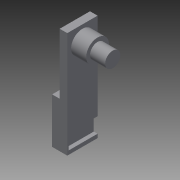
# Autodesk Inventor part: rotator_Base
Saved by Autodesk Inventor 2015 (Build 190159000, 159)
## iProperties
Created: 2015-04-10
Part Number: rotator_Base
Material: Generic
Document SubType Name: Modeling
Designer: WASHHSST
Density: 1 g/cm^3
Appearance: Default
Author: WASHHSST
Autodesk Inventor part; units mm, degrees
ref_plane "YZ Plane" through (0, 0, 0) normal (1, 0, 0) x (0, 1, 0)
ref_plane "XZ Plane" through (0, 0, 0) normal (0, 1, 0) x (-1, 0, 0)
ref_plane "XY Plane" through (0, 0, 0) normal (0, 0, 1) x (1, 0, 0)
sketch "Sketch1" plane through (0, 0, 0) normal (0, 1, 0) x (-1, 0, 0)
  line L0 (0, 0) -> (25.4, 0)
  line L1 (25.4, 0) -> (25.4, -50.8)
  line L2 (25.4, -50.8) -> (0, -50.8)
  line L3 (0, -50.8) -> (0, 0)
  dimension "d0" = 25.4
  dimension "d1" = 50.8
  constraints: 8 end point, 2 parallel, 1 horizontal, 1 perpendicular
  measures "d0" distance of L1.end L2.end
  measures "d1" distance of L0.end L1.end
extrude "Extrusion1" add sketch "Sketch1" along normal blind 25.4
sketch "Sketch2" plane through (0, 25.4, 0) normal (0, 1, 0) x (1, 0, 0)
  line L0 (-25.4, 0) -> (0, 0) projected
  line L1 (-12.7, 0) -> (-12.7, 50.8)
  line L2 (0, 50.8) -> (-25.4, 50.8) projected
  line L3 (0, 0) -> (0, 50.8) projected
  dimension "d4" = 12.7
  constraints: 2 end point, 2 midpoint, 1 vertical
  measures "d4" distance between parallel lines of L3 L1
extrude "Extrusion2" add sketch "Sketch2" along normal blind 101.6
sketch "Sketch3" plane through (0, 0, 0) normal (1, 0, 0) x (0, 0, -1)
  circle A0 centre (25.4, 101.6) radius 12.7
  line L0 (0, 0) -> (0, 127) projected
  line L1 (0, 127) -> (50.8, 127) projected
  dimension "d7" = 25.4
  dimension "d8" = 25.4
  dimension "d9" = 25.4
  constraints: 1 centre point
  measures "d7" diameter of A0
  measures "d8" distance from line of L0 A0.centre
  measures "d9" distance from line of L1 A0.centre
extrude "Extrusion3" add sketch "Sketch3" along normal blind 50.8
sketch "Sketch4" plane through (0, 0, 0) normal (0, -1, 0) x (1, 0, 0)
  line L0 (0, 0) -> (-25.4, 0)
  line L1 (-25.4, 0) -> (-25.4, -50.8)
  line L2 (-25.4, -50.8) -> (0, -50.8)
  line L3 (0, -50.8) -> (0, 0)
  constraints: 8 end point, 2 parallel, 1 horizontal, 1 perpendicular
extrude "Extrusion4" add sketch "Sketch4" along normal blind 50.8
sketch "Sketch6" plane through (-12.7, 25.4, -50.8) normal (0, 0, -1) x (-1, 0, 0)
  line L0 (-12.7, -76.2) -> (-12.7, -69.85)
  line L1 (-12.7, 101.6) -> (-12.7, -76.2) projected
  line L2 (-12.7, -69.85) -> (-6.35, -69.85)
  line L3 (-6.35, -69.85) -> (-6.35, -44.45)
  line L4 (-6.35, -44.45) -> (-12.7, -44.45)
  line L5 (-12.7, -76.2) -> (12.7, -76.2)
  line L6 (12.7, -76.2) -> (-12.7, -76.2) projected
  line L7 (12.7, -76.2) -> (12.7, -69.85)
  line L8 (12.7, 0) -> (12.7, -76.2) projected
  line L9 (12.7, -69.85) -> (6.35, -69.85)
  line L10 (6.35, -69.85) -> (6.35, -44.45)
  line L11 (6.35, -44.45) -> (12.7, -44.45)
  point P0 (-12.7, -25.4)
  dimension "d15" = 6.35
  dimension "d16" = 6.35
  dimension "d17" = 25.4
  dimension "d18" = 6.35
  dimension "d19" = 6.35
  dimension "d20" = 25.4
  constraints: 18 end point, 5 perpendicular, 4 point on line, 1 collinear, 1 parallel
  measures "d15" distance of L0.start L0.end
  measures "d16" distance of L0.end L2.end
  measures "d17" distance of L2.end L3.end
  measures "d18" distance of L7.end L9.end
  measures "d19" distance between parallel lines of L5 L9
  measures "d20" distance between parallel lines of L9 L11
extrude "Extrusion5" cut sketch "Sketch6" against normal blind 50.8
sketch "Sketch7" plane through (-12.7, 127, 0) normal (0, 0, 1) x (1, 0, 0)
  line L0 (-12.7, -177.8) -> (12.7, -177.8)
  line L1 (12.7, -177.8) -> (12.7, -146.05)
  line L2 (12.7, -146.05) -> (-12.7, -146.05)
  line L3 (-12.7, -146.05) -> (-12.7, -177.8)
  point P0 (12.7, -127)
  constraints: 8 end point, 2 parallel, 1 horizontal, 1 perpendicular
extrude "Extrusion6" add sketch "Sketch7" against normal blind 2.54
sketch "Sketch8" plane through (0, 127, 0) normal (1, 0, 0) x (0, 0, -1)
  circle A0 centre (25.4, -25.4) radius 19.05
  circle A1 centre (25.4, -25.4) radius 12.7 projected
  point P0 (0, -127)
  dimension "d25" = 38.1
  constraints: 1 centre point, 1 concentric
  measures "d25" diameter of A0
extrude "Extrusion7" add sketch "Sketch8" along normal blind 25.4
body "Solid1"
